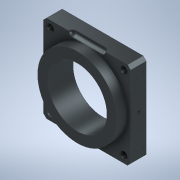
# Autodesk Inventor part: 0x001
Saved by Autodesk Inventor 2020 (Build 240168000, 168)
## iProperties
Created: 2024-01-28
Part Number: 0x001
Material: Iron, Cast
Document SubType Name: Modeling
Designer: ThorLabs
Density: 7.15 g/cm^3
Appearance: Iron Gray
Mass: 361.322 g
Surface Area: 156.808 cm^2
Volume: 50.5346 cm^3
Project: Motorized Rotator Mount
Description: Optical Mount
Engineer: ThorLabs
Author: Scott Bricker
Title: Optical Mount
Comments: Re-modeled replica of ThorLabs LCRM2_M for modeling purposes.
Revision Number: v1.0
Autodesk Inventor part; units mm, degrees
ref_plane "YZ Plane" through (0, 0, 0) normal (1, 0, 0) x (0, 1, 0)
ref_plane "XZ Plane" through (0, 0, 0) normal (0, 1, 0) x (-1, 0, 0)
ref_plane "XY Plane" through (0, 0, 0) normal (0, 0, 1) x (1, 0, 0)
sketch "Sketch1" plane through (0, 0, 0) normal (0, 0, 1) x (1, 0, 0)
  line L0 (0, 0) -> (71.1, 0)
  line L1 (71.1, 0) -> (71.1, 71.1)
  line L2 (71.1, 71.1) -> (0, 71.1)
  line L3 (0, 71.1) -> (0, 0)
  circle A0 centre (35.55, 35.55) radius 24.15
  dimension "d0" = 71.1
  dimension "d1" = 71.1
  dimension "d2" = 48.3
  constraints: 8 end point, 2 perpendicular, 1 centre point, 1 horizontal, 1 parallel
  measures "d0" distance of L0.start L0.end
  measures "d1" distance of L0.end L1.end
  measures "d2" diameter of A0
extrude "Extrusion1" add sketch "Sketch1" along normal blind 12.7
sketch "Sketch2" plane through (0, 0, 12.7) normal (0, 0, 1) x (1, 0, 0)
  line L0 (71.1, 71.1) -> (0, 71.1) projected
  line L1 (0, 71.1) -> (0, 0) projected
  line L2 (0, 0) -> (71.1, 0) projected
  line L3 (71.1, 0) -> (71.1, 71.1) projected
  circle A0 centre (35.55, 35.55) radius 24.15 projected
  circle A1 centre (35.55, 35.55) radius 24.15
  circle A2 centre (35.55, 35.55) radius 32.4
  dimension "d5" = 64.8
  constraints: 2 centre point, 2 coincident
  measures "d5" diameter of A2
extrude "Extrusion2" add sketch "Sketch2" along normal blind 7.9 contours A2
sketch "Sketch3" plane through (0, 71.1, 0) normal (0, 1, 0) x (1, 0, 0)
  line L0 (71.1, 0) -> (0, 0) projected
  line L1 (0, 0) -> (0, -12.7) projected
  line L2 (71.1, -12.7) -> (0, -12.7) projected
  line L3 (71.1, 0) -> (71.1, -12.7) projected
  line L4 (71.1, 0) -> (71.1, -12.7) projected
  line L5 (71.1, -12.7) -> (35.55, -12.7)
  line L6 (0, -12.7) -> (71.1, -12.7) projected
  line L7 (35.55, -12.7) -> (20.55, -12.7)
  line L8 (20.55, -12.7) -> (23.7, -12.7)
  arc A0 (23.7, -9.55) -> (20.55, -12.7) centre (23.7, -12.7) ccw
  line L9 (35.55, -12.7) -> (47.4, -12.7)
  arc A1 (50.55, -12.7) -> (47.4, -9.55) centre (47.4, -12.7) ccw
  line L10 (47.4, -9.55) -> (23.7, -9.55)
  dimension "d8" = 35.55
  dimension "d9" = 15
  dimension "d10" = 3.15
  dimension "d11" = 11.85
  dimension "d12" = 6.3
  constraints: 10 end point, 4 point on circle, 4 point on line, 2 centre point, 2 coincident, 2 tangent, 1 midpoint
  measures "d8" distance of L2.start L5.end
  measures "d9" distance of L7.end L5.end
  measures "d10" distance of L7.end L8.end
  measures "d11" distance of L5.end L9.end
  measures "d12" diameter of A1
revolve "Revolution1" cut sketch "Sketch3" angle 360 about axis through (71.1, 71.1, 12.7) along (-1, 0, 0) contours L2 A0 L10 A1
sketch "Sketch4" plane through (0, 0, 12.7) normal (0, 0, 1) x (1, 0, 0)
  arc A0 (20.55, 71.1) -> (23.7, 67.95) centre (23.7, 71.1) ccw projected
  line L0 (20.55, 71.1) -> (0, 71.1) projected
  line L1 (0, 71.1) -> (0, 0) projected
  line L2 (0, 0) -> (71.1, 0) projected
  line L3 (71.1, 0) -> (71.1, 71.1) projected
  line L4 (71.1, 71.1) -> (50.55, 71.1) projected
  arc A1 (47.4, 67.95) -> (50.55, 71.1) centre (47.4, 71.1) ccw projected
  line L5 (47.4, 67.95) -> (35.55, 67.95) projected
  circle A2 centre (35.55, 35.55) radius 32.4 projected
  line L6 (35.55, 67.95) -> (23.7, 67.95) projected
  line L7 (35.55, 35.55) -> (65.55, 35.55)
  line L8 (65.55, 35.55) -> (65.55, 65.55)
  line L9 (65.55, 65.55) -> (5.55, 65.55)
  line L10 (5.55, 65.55) -> (5.55, 5.55)
  line L11 (5.55, 5.55) -> (65.55, 5.55)
  circle A3 centre (65.55, 65.55) radius 3
  circle A4 centre (5.55, 65.55) radius 3
  circle A5 centre (5.55, 5.55) radius 3
  circle A6 centre (65.55, 5.55) radius 3
  dimension "d14" = 30
  dimension "d15" = 30
  dimension "d16" = 60
  dimension "d17" = 60
  dimension "d18" = 60
  dimension "d19" = 6
  dimension "d20" = 6
  dimension "d21" = 6
  dimension "d22" = 6
  constraints: 10 end point, 4 centre point, 4 coincident, 3 perpendicular, 1 horizontal, 1 point on line, 1 vertical alignment
  measures "d14" distance of L7.start L7.end
  measures "d15" distance of L7.end L8.end
  measures "d16" distance of L8.end L9.end
  measures "d17" distance of L9.end L10.end
  measures "d18" distance of L10.end L11.end
  measures "d19" diameter of A3
  measures "d20" diameter of A4
  measures "d21" diameter of A5
  measures "d22" diameter of A6
extrude "Extrusion3" cut sketch "Sketch4" against normal blind 12.7 contours A6 | A3 L8 L9 | L9 L8 A3 | A4 L10 L9 | L9 L10 A4 | A5 L11 L10 | L10 L11 A5
sketch "Sketch5" plane through (71.1, 0, 0) normal (1, 0, 0) x (0, 0, -1)
  line L0 (0, 0) -> (0, 71.1) projected
  line L1 (0, 71.1) -> (-12.7, 71.1) projected
  line L2 (-12.7, 0) -> (-12.7, 71.1) projected
  line L3 (0, 0) -> (-12.7, 0) projected
  line L4 (-12.7, 71.1) -> (-12.7, 0) projected
  line L5 (-12.7, 35.55) -> (-6.35, 35.55)
  circle A0 centre (-6.35, 35.55) radius 1
  line L6 (-6.35, 35.55) -> (-9.525, 35.55)
  line L7 (-9.525, 35.55) -> (-9.525, 65.55)
  line L8 (-9.525, 65.55) -> (-9.525, 61.97)
  line L9 (-9.525, 65.55) -> (-3.175, 65.55)
  line L10 (-3.175, 65.55) -> (-3.175, 5.55)
  line L11 (-3.175, 5.55) -> (-3.175, 9.13)
  line L12 (-3.175, 9.13) -> (-9.525, 9.13)
  circle A1 centre (-9.525, 9.13) radius 0.65
  circle A2 centre (-3.175, 9.13) radius 0.65
  circle A3 centre (-9.525, 61.97) radius 0.65
  circle A4 centre (-3.175, 61.97) radius 0.65
  line L13 (-9.525, 61.97) -> (-3.175, 61.97)
  dimension "d25" = 6.35
  dimension "d26" = 2
  dimension "d37" = 3.175
  dimension "d38" = 30
  dimension "d39" = 3.58
  dimension "d40" = 6.35
  dimension "d41" = 60
  dimension "d42" = 3.58
  dimension "d43" = 6.35
  dimension "d44" = 1.3
  dimension "d45" = 1.3
  dimension "d46" = 1.3
  dimension "d47" = 1.3
  dimension "d48" = 6.35
  constraints: 18 end point, 5 centre point, 4 coincident, 4 perpendicular, 3 point on line, 2 midpoint, 1 horizontal
  measures "d25" distance of L5.start L5.end
  measures "d26" diameter of A0
  measures "d37" distance of L6.start L6.end
  measures "d38" distance of L6.end L7.end
  measures "d39" distance of L7.end L8.end
  measures "d40" distance of L7.end L9.end
  measures "d41" distance of L9.end L10.end
  measures "d42" distance of L10.end L11.end
  measures "d43" distance of L11.end L12.end
  measures "d44" diameter of A1
  measures "d45" diameter of A2
  measures "d46" diameter of A3
  measures "d47" diameter of A4
  measures "d48" distance of L13.start L13.end
extrude "Extrusion4" cut sketch "Sketch5" against normal blind 4.75 contours A1 | A2 L10 | L10 L12 A2 | A3 L7 | L7 L13 A3 | A0 | L7 A3 L13 | L13 L10 A4 | A4 L10 L13 | A4 L10 | L10 A2 L12
sketch "Sketch6" plane through (0, 0, 0) normal (0, -1, 0) x (1, 0, 0)
  line L0 (0, 0) -> (71.1, 0) projected
  line L1 (71.1, 0) -> (71.1, 12.7) projected
  line L2 (0, 12.7) -> (71.1, 12.7) projected
  line L3 (0, 0) -> (0, 12.7) projected
  circle A0 centre (35.55, 6.35) radius 2
  dimension "d29" = 4
  constraints: 1 centre point
  measures "d29" diameter of A0
extrude "Extrusion5" cut sketch "Sketch6" against normal blind 6.1 contours A0
thread "Thread1" size "M4x0.7" class "6H" standard "ANSI Metric M Profile" full length
chamfer "Chamfer1" distance 2.55 angle 45 4 edges at (71.1, 71.1, 6.35) (71.1, 0, 6.35) (0, 71.1, 6.35) (0, 0, 6.35)
sketch "Sketch7" plane through (0, 2.55, 0) normal (-1, 0, 0) x (0, 0, 1)
  circle A0 centre (9.525, 6.58) radius 0.65 projected
  circle A1 centre (3.175, 6.58) radius 0.65 projected
  circle A2 centre (3.175, 59.42) radius 0.65 projected
  circle A3 centre (6.35, 33) radius 1 projected
  circle A4 centre (9.525, 59.42) radius 0.65 projected
  line L0 (0, 0) -> (12.7, 0) projected
  line L1 (0, 0) -> (0, 66) projected
  line L2 (12.7, 66) -> (0, 66) projected
  line L3 (12.7, 0) -> (12.7, 66) projected
  circle A5 centre (3.175, 59.42) radius 0.65
  circle A6 centre (9.525, 59.42) radius 0.65
  circle A7 centre (6.35, 33) radius 1
  circle A8 centre (3.175, 6.58) radius 0.65 projected
  circle A9 centre (3.175, 6.58) radius 0.65
  circle A10 centre (9.525, 6.58) radius 0.65
  point P0 (0, -2.55)
  dimension "d49" = 1.3
  dimension "d50" = 1.3
  dimension "d51" = 2
  dimension "d52" = 1.3
  dimension "d53" = 1.3
  constraints: 5 centre point, 5 coincident
  measures "d49" diameter of A5
  measures "d50" diameter of A6
  measures "d51" diameter of A7
  measures "d52" diameter of A9
  measures "d53" diameter of A10
extrude "Extrusion6" cut sketch "Sketch7" against normal blind 4.75 contours A0 | A1 | A2 | A3 | A4
body "Solid1"
